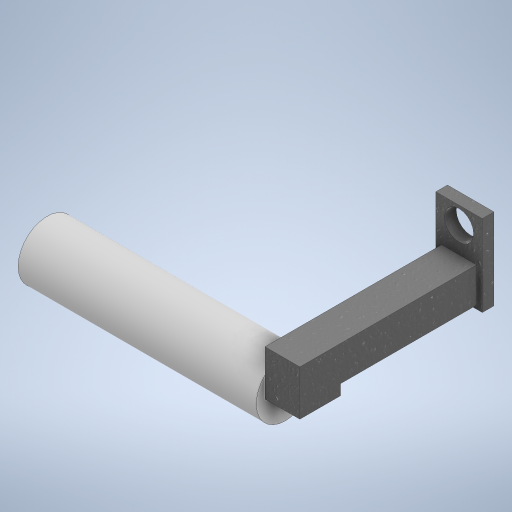
# Autodesk Inventor part: brazo
Saved by Autodesk Inventor 2023 (Build 270158030, 158C)
## iProperties
Created: 2022-05-25
Part Number: brazo
Material: Genérico
Document SubType Name: Modeling
Designer: isaac
Density: 1 g/cm^3
Appearance: Valor por defecto
Author: isaac
Autodesk Inventor part; units mm, degrees
ref_plane "YZ Plane" through (0, 0, 0) normal (1, 0, 0) x (0, 1, 0)
ref_plane "XZ Plane" through (0, 0, 0) normal (0, 1, 0) x (-1, 0, 0)
ref_plane "XY Plane" through (0, 0, 0) normal (0, 0, 1) x (1, 0, 0)
sketch "Boceto1" plane through (0, 0, 0) normal (0, 0, 1) x (1, 0, 0)
  line L0 (-20, 35) -> (20, 35)
  line L1 (20, 35) -> (20, -35)
  line L2 (20, -35) -> (-20, -35)
  line L3 (-20, -35) -> (-20, 35)
  circle A0 centre (0, 20) radius 12.5
  line L4 (-15, -2) -> (15, -2)
  line L5 (15, -2) -> (15, -32)
  line L6 (15, -32) -> (-15, -32)
  line L7 (-15, -32) -> (-15, -2)
  point P0 (0, 0)
  point P1 (0, 35)
  point P2 (-20, 0)
  point P3 (0, -2)
  point P4 (15, -17)
  point P5 (-15, -17)
  dimension "d0" = 70
  dimension "d1" = 25
  dimension "d2" = 20
  dimension "d3" = 40
  dimension "d8" = 30
  dimension "d9" = 30
  dimension "d10" = 3
  constraints: 16 end point, 5 midpoint, 4 parallel, 3 vertical alignment, 2 horizontal, 2 perpendicular, 1 centre point, 1 horizontal alignment
  measures "d0" distance between parallel lines of L2 L0
  measures "d1" diameter of A0
  measures "d2" distance of point (0, 0) A0.centre
  measures "d3" distance between parallel lines of L1 L3
  measures "d8" distance between parallel lines of L6 L4
  measures "d9" distance of point (15, -17) point (-15, -17)
  measures "d10" distance between parallel lines of L2 L6
extrude "Extrusión2" add sketch "Boceto1" along normal blind 10
extrude "Extrusión3" add sketch "Boceto1" along normal blind 162 contours L4 L5 L6 L7
sketch "Boceto2" plane through (-15, -32, 10) normal (0, -1, 0) x (1, 0, 0)
  line L0 (30, 0) -> (0, 0) construction
  line L1 (30, 0) -> (30, 152) construction
  line L2 (0, 152) -> (30, 152) construction
  line L3 (0, 0) -> (0, 152) construction
  line L4 (0, 0) -> (0, 152) projected
  line L5 (30, 0) -> (30, 152) projected
  line L6 (0, 152) -> (30, 152)
  line L7 (30, 152) -> (30, 117)
  line L8 (30, 117) -> (0, 117)
  line L9 (0, 117) -> (0, 152)
  point P0 (15, -10)
  point P1 (0, 117)
  dimension "d15" = 35
  constraints: 8 end point, 2 parallel, 1 horizontal, 1 perpendicular, 1 point on line
  measures "d15" distance of L6.end L7.end
extrude "Extrusión4" add sketch "Boceto2" along normal blind 9
sketch "Boceto3" plane through (-15, -32, 10) normal (-1, 0, 0) x (0, 0, 1)
  line L0 (117, -9) -> (152, -9) projected
  circle A0 centre (134.5, -9) radius 25
  point P0 (-10, 32)
  dimension "d18" = 50
  constraints: 1 centre point, 1 midpoint
  measures "d18" diameter of A0
extrude "Extrusión5" add sketch "Boceto3" along normal blind 205
